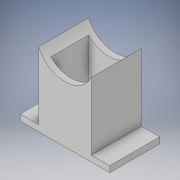
# Autodesk Inventor part: DPLX_P016_Spark_Gap_Camera_Shroud
Saved by Autodesk Inventor 2018 (Build 220112000, 112)
## iProperties
Created: 2018-06-12
Part Number: DPLX_P016_Spark_Gap_Camera_Shroud
Material: Generic
Document SubType Name: Modeling
Designer: DPLXuser
Density: 1 g/cm^3
Appearance: Default
Author: DPLXuser
Autodesk Inventor part; units mm, degrees
ref_plane "YZ Plane" through (0, 0, 0) normal (1, 0, 0) x (0, 1, 0)
ref_plane "XZ Plane" through (0, 0, 0) normal (0, 1, 0) x (-1, 0, 0)
ref_plane "XY Plane" through (0, 0, 0) normal (0, 0, 1) x (1, 0, 0)
sketch "Sketch1" plane through (0, 0, 0) normal (0, 1, 0) x (-1, 0, 0)
  line L0 (-13.7541, -13.0048) -> (13.7541, -13.0048)
  line L1 (13.7541, -13.0048) -> (13.7541, 13.0048)
  line L2 (13.7541, 13.0048) -> (-13.7541, 13.0048)
  line L3 (-13.7541, 13.0048) -> (-13.7541, -13.0048)
  line L4 (-13.7541, -13.0048) -> (13.7541, 13.0048) construction
  line L5 (13.7541, -13.0048) -> (-13.7541, 13.0048) construction
  point P0 (0, 0)
  dimension "d0" = 27.5082
  dimension "d1" = 26.0096
  constraints: 12 end point, 2 midpoint, 2 parallel, 1 horizontal, 1 perpendicular
  measures "d0" distance of L2.end L1.end
  measures "d1" distance of L1.end L0.end
extrude "Extrusion1" add sketch "Sketch1" along normal blind 39.1617
shell "Shell1" thickness 3.175 removed faces 2 at (4.5847, 0, -4.3349) at (4.5847, 39.1617, -4.3349)
sketch "Sketch2" plane through (0, 0, 0) normal (0, 0, 1) x (1, 0, 0)
  line L0 (0, 0) -> (0, 44.45)
  circle A0 centre (0, 44.45) radius 15.113
  dimension "d5" = 44.45
  dimension "d6" = 30.226
  constraints: 2 end point, 1 centre point, 1 coincident, 1 vertical
  measures "d5" distance of L0.start L0.end
  measures "d6" diameter of A0
extrude "Extrusion2" cut sketch "Sketch2" along normal mid plane 39.1617
sketch "Sketch3" plane through (13.7541, 0, 13.0048) normal (1, 0, 0) x (0, 0, -1)
  line L0 (26.0096, 0) -> (0, 0) projected
  line L1 (0, 0) -> (0, 38.1868) projected
  line L2 (26.0096, 0) -> (0, 0)
  line L3 (0, 0) -> (0, 3.175)
  line L4 (0, 3.175) -> (26.0096, 3.175)
  line L5 (26.0096, 3.175) -> (26.0096, 0)
  point P0 (13.0048, 0)
  dimension "d9" = 3.175
  constraints: 8 end point, 2 parallel, 1 horizontal, 1 perpendicular, 1 point on line
  measures "d9" distance of L2.end L3.end
extrude "Extrusion3" add sketch "Sketch3" along normal blind 9.525
sketch "Sketch4" plane through (-13.7541, 0, -13.0048) normal (-1, 0, 0) x (0, 0, 1)
  line L0 (26.0096, 3.175) -> (26.0096, 38.1868) projected
  line L1 (0, 0) -> (26.0096, 0)
  line L2 (26.0096, 0) -> (26.0096, 3.175)
  line L3 (26.0096, 3.175) -> (0, 3.175)
  line L4 (0, 3.175) -> (0, 0)
  point P0 (13.0048, 0)
  constraints: 8 end point, 2 parallel, 1 horizontal, 1 perpendicular
extrude "Extrusion4" add sketch "Sketch4" along normal blind 9.525
body "Solid1"
